Autodesk Fusion 360 part; units mm, degrees
(part 3 of 3)
  spline S561 degree 3 poles (81.8849, -47.0877) (82.1212, -46.8514) (82.4417, -46.7187) (82.7758, -46.7187) knots 0 0 0 0 1 1 1 1
  spline S562 degree 3 poles (112.4749, -35.3303) (112.8091, -35.3303) (113.1296, -35.4631) (113.3659, -35.6994) knots 0 0 0 0 1 1 1 1
  line L482 (113.7349, -36.5903) -> (113.7349, -36.5903)
  spline S563 degree 3 poles (51.3254, -35.9434) (51.2994, -35.4474) (50.8766, -35.0663) (50.3805, -35.0917) knots 0 0 0 0 1 1 1 1
  spline S564 degree 3 poles (43.0813, -29.5297) (43.3176, -29.2934) (43.6381, -29.1607) (43.9723, -29.1607) knots 0 0 0 0 1 1 1 1
  spline S565 degree 3 poles (54.9572, -31.105) (54.6231, -31.105) (54.3026, -30.9722) (54.0663, -30.7359) knots 0 0 0 0 1 1 1 1
  spline S566 degree 3 poles (51.5248, -30.1328) (51.5248, -30.6792) (51.3077, -31.2032) (50.9214, -31.5895) knots 0 0 0 0 1 1 1 1
  spline S567 degree 3 poles (43.0813, -31.3116) (42.845, -31.0753) (42.7123, -30.7549) (42.7123, -30.4207) knots 0 0 0 0 1 1 1 1
  spline S568 degree 3 poles (102.7091, -5.764) (103.0373, -6.0922) (103.2216, -6.5373) (103.2216, -7.0015) knots 0 0 0 0 1 1 1 1
  spline S569 degree 3 poles (88.275, -50.1347) (87.7287, -50.1347) (87.2047, -49.9176) (86.8184, -49.5313) knots 0 0 0 0 1 1 1 1
  spline S570 degree 3 poles (55.8482, -28.954) (56.0845, -29.1903) (56.2172, -29.5108) (56.2172, -29.845) knots 0 0 0 0 1 1 1 1
  spline S571 degree 3 poles (102.7091, -8.2389) (102.3809, -8.5671) (101.9358, -8.7515) (101.4716, -8.7515) knots 0 0 0 0 1 1 1 1
  spline S572 degree 3 poles (47.332, -19.1294) (47.358, -19.6254) (47.7808, -20.0065) (48.2768, -19.9811) knots 0 0 0 0 1 1 1 1
  spline S573 degree 3 poles (41.8226, -13.444) (41.8226, -13.1098) (41.9553, -12.7893) (42.1916, -12.553) knots 0 0 0 0 1 1 1 1
  spline S574 degree 3 poles (43.0826, -14.704) (42.7484, -14.704) (42.4279, -14.5712) (42.1916, -14.3349) knots 0 0 0 0 1 1 1 1
  spline S575 degree 3 poles (50.0317, -14.6128) (49.6454, -14.9991) (49.1214, -15.2161) (48.575, -15.2161) knots 0 0 0 0 1 1 1 1
  spline S576 degree 3 poles (71.5094, -50.5247) (71.3487, -50.2462) (71.0515, -50.0747) (70.73, -50.0747) knots 0 0 0 0 1 1 1 1
  line L483 (70.73, -50.0747) -> (69.42, -50.0747)
  spline S577 degree 3 poles (42.1916, -14.3349) (41.9553, -14.0986) (41.8226, -13.7782) (41.8226, -13.444) knots 0 0 0 0 1 1 1 1
  spline S578 degree 3 poles (48.575, -15.2161) (48.0287, -15.2161) (47.5047, -14.9991) (47.1184, -14.6128) knots 0 0 0 0 1 1 1 1
  spline S579 degree 3 poles (76.466, -45.9656) (76.2297, -46.2019) (75.9092, -46.3347) (75.575, -46.3347) knots 0 0 0 0 1 1 1 1
  spline S580 degree 3 poles (75.575, -46.3347) (75.2408, -46.3347) (74.9203, -46.2019) (74.684, -45.9656) knots 0 0 0 0 1 1 1 1
  spline S581 degree 3 poles (50.4357, -18.9667) (50.4097, -18.4707) (49.9868, -18.0896) (49.4908, -18.115) knots 0 0 0 0 1 1 1 1
  spline S582 degree 3 poles (55.3275, -12.8683) (55.3275, -13.2025) (55.1948, -13.5229) (54.9585, -13.7592) knots 0 0 0 0 1 1 1 1
  line L484 (49.585, -19.9125) -> (48.2768, -19.9811)
  spline S583 degree 3 poles (46.515, -13.1561) (46.515, -12.0184) (47.4373, -11.0961) (48.575, -11.0961) knots 0 0 0 0 1 1 1 1
  spline S584 degree 3 poles (50.0317, -11.6995) (50.418, -12.0858) (50.635, -12.6098) (50.635, -13.1561) knots 0 0 0 0 1 1 1 1
  spline S585 degree 3 poles (74.684, -45.9656) (74.4477, -45.7293) (74.315, -45.4088) (74.315, -45.0747) knots 0 0 0 0 1 1 1 1
  spline S586 degree 3 poles (70.73, -51.8747) (71.0515, -51.8747) (71.3487, -51.7031) (71.5094, -51.4247) knots 0 0 0 0 1 1 1 1
  spline S587 degree 3 poles (74.684, -44.1837) (74.9203, -43.9474) (75.2408, -43.8147) (75.575, -43.8147) knots 0 0 0 0 1 1 1 1
  spline S588 degree 3 poles (76.466, -44.1837) (76.7023, -44.42) (76.835, -44.7405) (76.835, -45.0747) knots 0 0 0 0 1 1 1 1
  spline S589 degree 3 poles (75.575, -43.8147) (75.9092, -43.8147) (76.2297, -43.9474) (76.466, -44.1837) knots 0 0 0 0 1 1 1 1
  spline S590 degree 3 poles (54.0675, -11.6083) (54.4017, -11.6083) (54.7222, -11.741) (54.9585, -11.9773) knots 0 0 0 0 1 1 1 1
  spline S591 degree 3 poles (43.0826, -12.184) (43.4168, -12.184) (43.7372, -12.3167) (43.9735, -12.553) knots 0 0 0 0 1 1 1 1
  line L485 (70.73, -51.8747) -> (69.42, -51.8747)
  spline S592 degree 3 poles (48.575, -11.0961) (49.1214, -11.0961) (49.6454, -11.3132) (50.0317, -11.6995) knots 0 0 0 0 1 1 1 1
  spline S593 degree 3 poles (53.1766, -13.7592) (52.9403, -13.5229) (52.8075, -13.2025) (52.8075, -12.8683) knots 0 0 0 0 1 1 1 1
  spline S594 degree 3 poles (53.1766, -11.9773) (53.4129, -11.741) (53.7333, -11.6083) (54.0675, -11.6083) knots 0 0 0 0 1 1 1 1
  spline S595 degree 3 poles (47.1184, -14.6128) (46.7321, -14.2264) (46.515, -13.7025) (46.515, -13.1561) knots 0 0 0 0 1 1 1 1
  spline S596 degree 3 poles (74.315, -45.0747) (74.315, -44.7405) (74.4477, -44.42) (74.684, -44.1837) knots 0 0 0 0 1 1 1 1
  line L486 (55.3275, -12.8683) -> (55.3275, -12.8683)
  spline S597 degree 3 poles (43.9735, -12.553) (44.2098, -12.7893) (44.3426, -13.1098) (44.3426, -13.444) knots 0 0 0 0 1 1 1 1
  spline S598 degree 3 poles (52.8075, -12.8683) (52.8075, -12.5341) (52.9403, -12.2136) (53.1766, -11.9773) knots 0 0 0 0 1 1 1 1
  spline S599 degree 3 poles (76.835, -45.0747) (76.835, -45.4088) (76.7023, -45.7293) (76.466, -45.9656) knots 0 0 0 0 1 1 1 1
  spline S600 degree 3 poles (68.6406, -50.5247) (68.4798, -50.8031) (68.4798, -51.1462) (68.6406, -51.4247) knots 0 0 0 0 1 1 1 1
  spline S601 degree 3 poles (72.135, -45.0747) (72.135, -45.621) (71.918, -46.145) (71.5316, -46.5313) knots 0 0 0 0 1 1 1 1
  spline S602 degree 3 poles (48.1826, -18.1836) (47.6867, -18.2101) (47.306, -18.6334) (47.332, -19.1294) knots 0 0 0 0 1 1 1 1
  spline S603 degree 3 poles (54.9585, -13.7592) (54.7222, -13.9955) (54.4017, -14.1283) (54.0675, -14.1283) knots 0 0 0 0 1 1 1 1
  line L487 (44.3426, -13.444) -> (44.3426, -13.444)
  spline S604 degree 3 poles (68.6406, -51.4247) (68.8013, -51.7031) (69.0985, -51.8747) (69.42, -51.8747) knots 0 0 0 0 1 1 1 1
  spline S605 degree 3 poles (69.42, -50.0747) (69.0985, -50.0747) (68.8013, -50.2462) (68.6406, -50.5247) knots 0 0 0 0 1 1 1 1
  spline S606 degree 3 poles (49.585, -19.9125) (50.081, -19.886) (50.4617, -19.4627) (50.4357, -18.9667) knots 0 0 0 0 1 1 1 1
  spline S607 degree 3 poles (71.5316, -46.5313) (71.1453, -46.9176) (70.6213, -47.1347) (70.075, -47.1347) knots 0 0 0 0 1 1 1 1
  spline S608 degree 3 poles (44.3426, -13.444) (44.3426, -13.7782) (44.2098, -14.0986) (43.9735, -14.3349) knots 0 0 0 0 1 1 1 1
  spline S609 degree 3 poles (68.015, -45.0747) (68.015, -43.9369) (68.9373, -43.0147) (70.075, -43.0147) knots 0 0 0 0 1 1 1 1
  spline S610 degree 3 poles (70.075, -47.1347) (69.5287, -47.1347) (69.0047, -46.9176) (68.6184, -46.5313) knots 0 0 0 0 1 1 1 1
  spline S611 degree 3 poles (54.9585, -11.9773) (55.1948, -12.2136) (55.3275, -12.5341) (55.3275, -12.8683) knots 0 0 0 0 1 1 1 1
  line L488 (72.135, -45.0747) -> (72.135, -45.0747)
  spline S612 degree 3 poles (65.835, -45.0747) (65.835, -45.4088) (65.7023, -45.7293) (65.466, -45.9656) knots 0 0 0 0 1 1 1 1
  spline S613 degree 3 poles (70.075, -43.0147) (70.6213, -43.0147) (71.1453, -43.2317) (71.5316, -43.618) knots 0 0 0 0 1 1 1 1
  spline S614 degree 3 poles (64.575, -46.3347) (64.2408, -46.3347) (63.9203, -46.2019) (63.684, -45.9656) knots 0 0 0 0 1 1 1 1
  spline S615 degree 3 poles (54.0675, -14.1283) (53.7333, -14.1283) (53.4129, -13.9955) (53.1766, -13.7592) knots 0 0 0 0 1 1 1 1
  spline S616 degree 3 poles (43.9735, -14.3349) (43.7372, -14.5712) (43.4168, -14.704) (43.0826, -14.704) knots 0 0 0 0 1 1 1 1
  spline S617 degree 3 poles (65.466, -45.9656) (65.2297, -46.2019) (64.9092, -46.3347) (64.575, -46.3347) knots 0 0 0 0 1 1 1 1
  spline S618 degree 3 poles (42.1916, -12.553) (42.4279, -12.3167) (42.7484, -12.184) (43.0826, -12.184) knots 0 0 0 0 1 1 1 1
  spline S619 degree 3 poles (71.5094, -51.4247) (71.6702, -51.1462) (71.6702, -50.8031) (71.5094, -50.5247) knots 0 0 0 0 1 1 1 1
  spline S620 degree 3 poles (68.6184, -46.5313) (68.232, -46.145) (68.015, -45.621) (68.015, -45.0747) knots 0 0 0 0 1 1 1 1
  spline S621 degree 3 poles (63.315, -45.0747) (63.315, -44.7405) (63.4477, -44.42) (63.684, -44.1837) knots 0 0 0 0 1 1 1 1
  spline S622 degree 3 poles (63.684, -45.9656) (63.4477, -45.7293) (63.315, -45.4088) (63.315, -45.0747) knots 0 0 0 0 1 1 1 1
  line L489 (49.4908, -18.115) -> (48.1826, -18.1836)
  line L490 (50.635, -13.1561) -> (50.635, -13.1561)
  line L491 (76.835, -45.0747) -> (76.835, -45.0747)
  spline S623 degree 3 poles (71.5316, -43.618) (71.918, -44.0043) (72.135, -44.5283) (72.135, -45.0747) knots 0 0 0 0 1 1 1 1
  spline S624 degree 3 poles (50.635, -13.1561) (50.635, -13.7025) (50.418, -14.2264) (50.0317, -14.6128) knots 0 0 0 0 1 1 1 1
  line L492 (65.835, -45.0747) -> (65.835, -45.0747)
  line L493 (110.7912, -73.1802) -> (111.0216, -73.8484)
  spline S625 degree 3 poles (63.684, -44.1837) (63.9203, -43.9474) (64.2408, -43.8147) (64.575, -43.8147) knots 0 0 0 0 1 1 1 1
  spline S626 degree 3 poles (3.6391, -67.1258) (4.4065, -69.4383) (6.4962, -71.0571) (8.9271, -71.2222) knots 0 0 0 0 1 1 1 1
  line L494 (116.1996, -81.9373) -> (119.0491, -76.0948)
  spline S627 degree 3 poles (118.8062, -6.1021) (83.6894, 2.7201) (46.8363, 1.8437) (12.1786, -8.6379) knots 0 0 0 0 1 1 1 1
  spline S628 degree 3 poles (118.1824, -90.992) (120.517, -91.6893) (123.0415, -90.9056) (124.5707, -89.0087) knots 0 0 0 0 1 1 1 1
  spline S629 degree 3 poles (65.466, -44.1837) (65.7023, -44.42) (65.835, -44.7405) (65.835, -45.0747) knots 0 0 0 0 1 1 1 1
  spline S630 degree 3 poles (138.6019, -30.79) (137.1962, -24.0467) (134.803, -17.5478) (131.4995, -11.5033) knots 0 0 0 0 1 1 1 1
  spline S631 degree 3 poles (64.575, -43.8147) (64.9092, -43.8147) (65.2297, -43.9474) (65.466, -44.1837) knots 0 0 0 0 1 1 1 1
  line L495 (115.2322, -66.3558) -> (114.1098, -68.657)
  line L496 (114.1098, -68.657) -> (113.6783, -68.4466)
  line L497 (111.2113, -79.5044) -> (110.0827, -81.8184)
  line L498 (115.3459, -81.5208) -> (116.1996, -81.9373)
  spline S632 degree 3 poles (124.5707, -89.0087) (128.8939, -83.6461) (132.402, -77.6748) (134.9814, -71.2878) knots 0 0 0 0 1 1 1 1
  spline S633 degree 3 poles (8.9271, -71.2222) (45.9666, -73.7356) (82.6109, -80.3665) (118.1824, -90.992) knots 0 0 0 0 1 1 1 1
  spline S634 degree 3 poles (97.4738, -79.183) (97.9614, -79.2773) (98.4333, -78.9586) (98.5281, -78.4711) knots 0 0 0 0 1 1 1 1
  spline S635 degree 3 poles (118.1954, -75.6788) (117.8944, -75.4783) (117.6795, -75.1722) (117.5933, -74.8209) knots 0 0 0 0 1 1 1 1
  line L499 (117.7292, -73.7822) -> (118.4305, -72.3441)
  line L500 (110.0827, -81.8184) -> (114.2168, -83.8348)
  line L501 (118.4305, -72.3441) -> (118.0383, -71.0961)
  spline S636 degree 3 poles (117.5933, -74.8209) (117.507, -74.4699) (117.5555, -74.0992) (117.7292, -73.7822) knots 0 0 0 0 1 1 1 1
  line L502 (114.2168, -83.8348) -> (115.3459, -81.5208)
  spline S637 degree 3 poles (139.7972, -51.3076) (140.4104, -44.4469) (140.0076, -37.5332) (138.6019, -30.79) knots 0 0 0 0 1 1 1 1
  spline S638 degree 3 poles (98.5281, -78.4711) (98.6228, -77.9835) (98.3047, -77.5113) (97.8172, -77.4161) knots 0 0 0 0 1 1 1 1
  line L503 (111.0216, -73.8484) -> (111.9203, -74.2871)
  spline S639 degree 3 poles (112.2014, -74.701) (112.2073, -74.7888) (112.1896, -74.8766) (112.1503, -74.9553) knots 0 0 0 0 1 1 1 1
  line L504 (112.1503, -74.9553) -> (110.1778, -79)
  spline S640 degree 3 poles (8.6506, -11.5033) (-0.664, -28.546) (-2.4792, -48.6926) (3.6391, -67.1258) knots 0 0 0 0 1 1 1 1
  spline S641 degree 3 poles (134.9814, -71.2878) (137.561, -64.901) (139.1837, -58.1684) (139.7972, -51.3076) knots 0 0 0 0 1 1 1 1
  line L505 (112.9833, -68.6859) -> (110.7912, -73.1802)
  spline S642 degree 3 poles (131.4995, -11.5033) (130.7448, -10.1225) (129.4778, -9.0934) (127.9715, -8.6379) knots 0 0 0 0 1 1 1 1
  line L506 (110.1778, -79) -> (111.2113, -79.5044)
  line L507 (119.3664, -68.3727) -> (115.2322, -66.3558)
  line L508 (115.2322, -66.3558) -> (115.2322, -66.3558)
  spline S643 degree 3 poles (112.1172, -74.4556) (112.1666, -74.5284) (112.1957, -74.6132) (112.2014, -74.701) knots 0 0 0 0 1 1 1 1
  line L509 (113.6783, -68.4466) -> (112.9833, -68.6859)
  line L510 (119.0491, -76.0948) -> (118.1954, -75.6788)
  spline S644 degree 3 poles (111.9203, -74.2871) (111.9997, -74.3248) (112.0677, -74.3829) (112.1172, -74.4556) knots 0 0 0 0 1 1 1 1
  spline S645 degree 3 poles (12.1786, -8.6379) (10.6723, -9.0934) (9.4054, -10.1225) (8.6506, -11.5033) knots 0 0 0 0 1 1 1 1
  line L511 (118.0383, -71.0961) -> (119.3664, -68.3727)
  spline S646 degree 3 poles (74.315, -11.0747) (74.315, -10.7405) (74.4477, -10.42) (74.684, -10.1837) knots 0 0 0 0 1 1 1 1
  line L512 (72.135, -11.0747) -> (72.135, -11.0747)
  spline S647 degree 3 poles (40.9202, -28.6515) (41.5169, -28.6515) (42.0892, -28.8885) (42.5112, -29.3105) knots 0 0 0 0 1 1 1 1
  spline S648 degree 3 poles (59.9702, -9.6015) (60.5669, -9.6015) (61.1392, -9.8385) (61.5612, -10.2605) knots 0 0 0 0 1 1 1 1
  line L513 (73.095, -19.3947) -> (73.095, -19.8747)
  line L514 (65.835, -11.0747) -> (65.835, -11.0747)
  spline S649 degree 3 poles (57.7202, -11.8515) (57.7202, -11.2547) (57.9573, -10.6824) (58.3792, -10.2605) knots 0 0 0 0 1 1 1 1
  line L515 (118.8062, -6.1023) -> (117.075, -12.3447)
  spline S650 degree 3 poles (63.684, -11.9656) (63.4477, -11.7293) (63.315, -11.4088) (63.315, -11.0747) knots 0 0 0 0 1 1 1 1
  spline S651 degree 3 poles (70.075, -9.0147) (70.6213, -9.0147) (71.1453, -9.2317) (71.5316, -9.618) knots 0 0 0 0 1 1 1 1
  spline S652 degree 3 poles (65.835, -11.0747) (65.835, -11.4088) (65.7023, -11.7293) (65.466, -11.9656) knots 0 0 0 0 1 1 1 1
  spline S653 degree 3 poles (70.075, -13.1347) (69.5287, -13.1347) (69.0047, -12.9176) (68.6184, -12.5313) knots 0 0 0 0 1 1 1 1
  spline S654 degree 3 poles (63.315, -11.0747) (63.315, -10.7405) (63.4477, -10.42) (63.684, -10.1837) knots 0 0 0 0 1 1 1 1
  line L516 (86.2116, -49.5825) -> (86.2116, -52.9465)
  spline S655 degree 3 poles (43.1702, -30.9015) (43.1702, -31.4982) (42.9331, -32.0705) (42.5112, -32.4925) knots 0 0 0 0 1 1 1 1
  spline S656 degree 3 poles (39.3292, -32.4925) (38.9073, -32.0705) (38.6702, -31.4982) (38.6702, -30.9015) knots 0 0 0 0 1 1 1 1
  line L517 (70.73, -17.8747) -> (69.42, -17.8747)
  spline S657 degree 3 poles (61.5612, -10.2605) (61.9831, -10.6824) (62.2202, -11.2547) (62.2202, -11.8515) knots 0 0 0 0 1 1 1 1
  line L518 (43.1702, -30.9015) -> (43.1702, -30.9015)
  line L519 (78.8459, -52.9465) -> (78.8459, -49.5825)
  line L520 (73.095, -19.8747) -> (75.655, -19.8747)
  spline S658 degree 3 poles (58.3792, -10.2605) (58.8012, -9.8385) (59.3735, -9.6015) (59.9702, -9.6015) knots 0 0 0 0 1 1 1 1
  line L521 (68.575, -27.5747) -> (68.575, -26.6247)
  line L522 (67.075, -20.3747) -> (67.075, -19.3747)
  spline S659 degree 3 poles (71.5316, -9.618) (71.918, -10.0043) (72.135, -10.5283) (72.135, -11.0747) knots 0 0 0 0 1 1 1 1
  line L523 (62.075, -27.5747) -> (62.075, -26.6247)
  spline S660 degree 3 poles (59.9702, -14.1015) (59.3735, -14.1015) (58.8012, -13.8644) (58.3792, -13.4425) knots 0 0 0 0 1 1 1 1
  spline S661 degree 3 poles (75.575, -9.8147) (75.9092, -9.8147) (76.2297, -9.9474) (76.466, -10.1837) knots 0 0 0 0 1 1 1 1
  spline S662 degree 3 poles (68.6184, -12.5313) (68.232, -12.145) (68.015, -11.621) (68.015, -11.0747) knots 0 0 0 0 1 1 1 1
  line L524 (86.2116, -52.9465) -> (78.8459, -52.9465)
  spline S663 degree 3 poles (74.684, -10.1837) (74.9203, -9.9474) (75.2408, -9.8147) (75.575, -9.8147) knots 0 0 0 0 1 1 1 1
  spline S664 degree 3 poles (65.466, -11.9656) (65.2297, -12.2019) (64.9092, -12.3347) (64.575, -12.3347) knots 0 0 0 0 1 1 1 1
  line L525 (78.8459, -49.5825) -> (86.2116, -49.5825)
  spline S665 degree 3 poles (70.075, -25.3747) (69.3264, -25.3389) (68.6749, -25.8819) (68.575, -26.6247) knots 0 0 0 0 1 1 1 1
  line L526 (62.2202, -11.8515) -> (62.2202, -11.8515)
  spline S666 degree 3 poles (76.466, -10.1837) (76.7023, -10.42) (76.835, -10.7405) (76.835, -11.0747) knots 0 0 0 0 1 1 1 1
  line L527 (126.0175, -14.8246) -> (127.7516, -8.5716)
  spline S667 degree 3 poles (64.575, -12.3347) (64.2408, -12.3347) (63.9203, -12.2019) (63.684, -11.9656) knots 0 0 0 0 1 1 1 1
  spline S668 degree 3 poles (64.575, -9.8147) (64.9092, -9.8147) (65.2297, -9.9474) (65.466, -10.1837) knots 0 0 0 0 1 1 1 1
  spline S669 degree 3 poles (63.684, -10.1837) (63.9203, -9.9474) (64.2408, -9.8147) (64.575, -9.8147) knots 0 0 0 0 1 1 1 1
  spline S670 degree 3 poles (65.466, -10.1837) (65.7023, -10.42) (65.835, -10.7405) (65.835, -11.0747) knots 0 0 0 0 1 1 1 1
  spline S671 degree 3 poles (61.5612, -13.4425) (61.1392, -13.8644) (60.5669, -14.1015) (59.9702, -14.1015) knots 0 0 0 0 1 1 1 1
  spline S672 degree 3 poles (38.6702, -30.9015) (38.6702, -30.3047) (38.9073, -29.7324) (39.3292, -29.3105) knots 0 0 0 0 1 1 1 1
  spline S673 degree 3 poles (66.575, -20.8747) (66.708, -20.876) (66.836, -20.8238) (66.9301, -20.7297) knots 0 0 0 0 1 1 1 1
  spline S674 degree 3 poles (39.3292, -29.3105) (39.7512, -28.8885) (40.3235, -28.6515) (40.9202, -28.6515) knots 0 0 0 0 1 1 1 1
  spline S675 degree 3 poles (71.5316, -12.5313) (71.1453, -12.9176) (70.6213, -13.1347) (70.075, -13.1347) knots 0 0 0 0 1 1 1 1
  spline S676 degree 3 poles (40.9202, -33.1515) (40.3235, -33.1515) (39.7512, -32.9144) (39.3292, -32.4925) knots 0 0 0 0 1 1 1 1
  line L528 (117.075, -12.3447) -> (126.0175, -14.8246)
  line L529 (68.575, -27.5747) -> (62.075, -27.5747)
  spline S677 degree 3 poles (42.5112, -32.4925) (42.0892, -32.9144) (41.5169, -33.1515) (40.9202, -33.1515) knots 0 0 0 0 1 1 1 1
  spline S678 degree 3 poles (42.5112, -29.3105) (42.9331, -29.7324) (43.1702, -30.3047) (43.1702, -30.9015) knots 0 0 0 0 1 1 1 1
  spline S679 degree 3 poles (72.135, -11.0747) (72.135, -11.621) (71.918, -12.145) (71.5316, -12.5313) knots 0 0 0 0 1 1 1 1
  spline S680 degree 3 poles (66.9301, -20.7297) (67.0241, -20.6356) (67.0764, -20.5077) (67.075, -20.3747) knots 0 0 0 0 1 1 1 1
  line L530 (72.575, -18.8747) -> (73.095, -19.3947)
  spline S681 degree 3 poles (62.2202, -11.8515) (62.2202, -12.4482) (61.9831, -13.0205) (61.5612, -13.4425) knots 0 0 0 0 1 1 1 1
  line L531 (62.075, -22.0247) -> (62.075, -20.8747)
  spline S682 degree 3 poles (58.3792, -13.4425) (57.9573, -13.0205) (57.7202, -12.4482) (57.7202, -11.8515) knots 0 0 0 0 1 1 1 1
  line L532 (76.835, -11.0747) -> (76.835, -11.0747)
  spline S683 degree 3 poles (68.015, -11.0747) (68.015, -9.9369) (68.9373, -9.0147) (70.075, -9.0147) knots 0 0 0 0 1 1 1 1
  spline S684 degree 3 poles (104.9284, -54.8447) (104.542, -54.4584) (104.325, -53.9344) (104.325, -53.388) knots 0 0 0 0 1 1 1 1
  spline S685 degree 3 poles (100.8883, -54.4561) (100.1925, -54.4561) (99.6283, -53.892) (99.6283, -53.1961) knots 0 0 0 0 1 1 1 1
  spline S686 degree 3 poles (100.8883, -51.9361) (101.2225, -51.9361) (101.543, -52.0688) (101.7793, -52.3051) knots 0 0 0 0 1 1 1 1
  spline S687 degree 3 poles (107.7325, -59.3387) (107.7498, -58.8422) (107.3616, -58.4255) (106.8651, -58.4079) knots 0 0 0 0 1 1 1 1
  line L533 (62.075, -20.8747) -> (66.575, -20.8747)
  spline S688 degree 3 poles (68.6406, -17.4247) (68.8013, -17.7031) (69.0985, -17.8747) (69.42, -17.8747) knots 0 0 0 0 1 1 1 1
  line L534 (71.675, -25.3747) -> (70.075, -25.3747)
  line L535 (75.655, -24.4747) -> (75.655, -19.8747)
  spline S689 degree 3 poles (76.466, -11.9656) (76.2297, -12.2019) (75.9092, -12.3347) (75.575, -12.3347) knots 0 0 0 0 1 1 1 1
  spline S690 degree 3 poles (71.5094, -17.4247) (71.6702, -17.1462) (71.6702, -16.8031) (71.5094, -16.5247) knots 0 0 0 0 1 1 1 1
  line L536 (67.575, -18.8747) -> (72.575, -18.8747)
  line L537 (72.625, -24.4747) -> (71.675, -25.3747)
  spline S691 degree 3 poles (71.5094, -16.5247) (71.3487, -16.2462) (71.0515, -16.0747) (70.73, -16.0747) knots 0 0 0 0 1 1 1 1
  spline S692 degree 3 poles (74.684, -11.9656) (74.4477, -11.7293) (74.315, -11.4088) (74.315, -11.0747) knots 0 0 0 0 1 1 1 1
  line L538 (70.73, -16.0747) -> (69.42, -16.0747)
  line L539 (104.7873, -73.4324) -> (104.7873, -73.4324)
  spline S693 degree 3 poles (100.1883, -72.3829) (100.1883, -73.5206) (99.266, -74.4429) (98.1283, -74.4429) knots 0 0 0 0 1 1 1 1
  spline S694 degree 3 poles (96.6717, -73.8396) (96.2853, -73.4533) (96.0683, -72.9293) (96.0683, -72.3829) knots 0 0 0 0 1 1 1 1
  line L540 (62.075, -26.6247) -> (59.5, -26.6247)
  spline S695 degree 3 poles (103.5273, -72.1724) (103.8614, -72.1724) (104.1819, -72.3051) (104.4182, -72.5414) knots 0 0 0 0 1 1 1 1
  spline S696 degree 3 poles (98.1283, -74.4429) (97.582, -74.4429) (97.058, -74.2259) (96.6717, -73.8396) knots 0 0 0 0 1 1 1 1
  line L541 (100.1883, -72.3829) -> (100.1883, -72.3829)
  spline S697 degree 3 poles (106.8023, -60.2068) (107.2988, -60.2237) (107.7152, -59.8352) (107.7325, -59.3387) knots 0 0 0 0 1 1 1 1
  line L542 (59.5, -22.0247) -> (62.075, -22.0247)
  spline S698 degree 3 poles (105.5559, -58.3621) (105.0594, -58.3451) (104.643, -58.7337) (104.6257, -59.2302) knots 0 0 0 0 1 1 1 1
  spline S699 degree 3 poles (108.445, -53.388) (108.445, -53.9344) (108.228, -54.4584) (107.8416, -54.8447) knots 0 0 0 0 1 1 1 1
  spline S700 degree 3 poles (104.6257, -59.2302) (104.6083, -59.7267) (104.9966, -60.1433) (105.4931, -60.161) knots 0 0 0 0 1 1 1 1
  line L543 (106.8023, -60.2068) -> (105.4931, -60.161)
  spline S701 degree 3 poles (107.8416, -54.8447) (107.4553, -55.231) (106.9313, -55.448) (106.385, -55.448) knots 0 0 0 0 1 1 1 1
  spline S702 degree 3 poles (104.9284, -51.9314) (105.3147, -51.5451) (105.8387, -51.328) (106.385, -51.328) knots 0 0 0 0 1 1 1 1
  spline S703 degree 3 poles (106.385, -51.328) (106.9313, -51.328) (107.4553, -51.5451) (107.8416, -51.9314) knots 0 0 0 0 1 1 1 1
  spline S704 degree 3 poles (76.835, -11.0747) (76.835, -11.4088) (76.7023, -11.7293) (76.466, -11.9656) knots 0 0 0 0 1 1 1 1
  line L544 (108.445, -53.388) -> (108.445, -53.388)
  spline S705 degree 3 poles (101.7793, -54.087) (101.543, -54.3233) (101.2225, -54.4561) (100.8883, -54.4561) knots 0 0 0 0 1 1 1 1
  spline S706 degree 3 poles (104.325, -53.388) (104.325, -52.8417) (104.542, -52.3177) (104.9284, -51.9314) knots 0 0 0 0 1 1 1 1
  spline S707 degree 3 poles (70.73, -17.8747) (71.0515, -17.8747) (71.3487, -17.7031) (71.5094, -17.4247) knots 0 0 0 0 1 1 1 1
  spline S708 degree 3 poles (75.575, -12.3347) (75.2408, -12.3347) (74.9203, -12.2019) (74.684, -11.9656) knots 0 0 0 0 1 1 1 1
  spline S709 degree 3 poles (102.6363, -72.5414) (102.8726, -72.3051) (103.1931, -72.1724) (103.5273, -72.1724) knots 0 0 0 0 1 1 1 1
  line L545 (67.075, -19.3747) -> (67.575, -18.8747)
  line L546 (75.655, -24.4747) -> (72.625, -24.4747)
  spline S710 degree 3 poles (96.6717, -70.9263) (97.058, -70.54) (97.582, -70.3229) (98.1283, -70.3229) knots 0 0 0 0 1 1 1 1
  line L547 (59.5, -26.6247) -> (59.5, -22.0247)
  spline S711 degree 3 poles (98.1283, -70.3229) (99.266, -70.3229) (100.1883, -71.2452) (100.1883, -72.3829) knots 0 0 0 0 1 1 1 1
  line L548 (106.8651, -58.4079) -> (105.5559, -58.3621)
  spline S712 degree 3 poles (106.385, -55.448) (105.8387, -55.448) (105.3147, -55.231) (104.9284, -54.8447) knots 0 0 0 0 1 1 1 1
  spline S713 degree 3 poles (107.8416, -51.9314) (108.228, -52.3177) (108.445, -52.8417) (108.445, -53.388) knots 0 0 0 0 1 1 1 1
  spline S714 degree 3 poles (69.42, -16.0747) (69.0985, -16.0747) (68.8013, -16.2462) (68.6406, -16.5247) knots 0 0 0 0 1 1 1 1
  spline S715 degree 3 poles (104.4182, -72.5414) (104.6545, -72.7777) (104.7873, -73.0982) (104.7873, -73.4324) knots 0 0 0 0 1 1 1 1
  spline S716 degree 3 poles (102.1483, -53.1961) (102.1483, -53.5303) (102.0156, -53.8508) (101.7793, -54.087) knots 0 0 0 0 1 1 1 1
  spline S717 degree 3 poles (68.6406, -16.5247) (68.4798, -16.8031) (68.4798, -17.1462) (68.6406, -17.4247) knots 0 0 0 0 1 1 1 1
  spline S718 degree 3 poles (96.0683, -72.3829) (96.0683, -71.8366) (96.2853, -71.3126) (96.6717, -70.9263) knots 0 0 0 0 1 1 1 1
extrude "Extrude2" add sketch "Sketch1" along normal blind 1 from surface at 3 contours S0 S14 S23 S43 S179 S180 L362 S181 L365 L366 L367 L368 L372 L381 L382 L383 L384 L385 L390 L394 L396 L398 L399 L400 L403 S710 S718 | S7 S44 L255 L258 L260 L262 L263 L264 L265 L266 L267 L268 L270 L271 L276 L277 L380 S194 L388 L389 L391 S217 S224 S686 S702 S706 | S18 S22 S50 S233 S237 L406 L408 L409 L410 L412 L413 L414 L415 L417 L418 S250 L422 L423 L424 L425 L426 L428 S278 S290 S299 S314 S318 | S25 S32 S37 L8 L10 L13 L16 L34 L35 L39 L40 L41 L42 L43 L44 L48 L49 L54 L56 L59 L65 S373 S379 S380 S383 S396 | L14 S51 L17 L18 L25 L27 L29 L30 L31 L32 L36 L45 S59 L55 L57 L58 L60 S61 L62 L63 L64 S265 S267 S297 S310 S316 | L15 L19 L20 L21 L22 L23 L26 L28 L33 L37 L38 L46 L47 L50 L51 L52 S57 S58 L53 S60 L93 S208 S209 S210 S220 S221 | S62 L66 L67 S63 L68 L69 L70 S65 L72 L73 L74 L75 L80 L81 L89 L94 L95 L98 L99 L101 L106 S464 S471 S494 S504 S511 S517 | L78 L79 L84 L85 L86 S74 L87 L88 L90 L91 L92 S76 L96 S77 L100 L102 L103 L104 L105 L116 L142 L154 S469 S473 S478 S479 S500 S507 | S79 L111 S82 L112 L113 L114 S83 L115 L117 S87 L119 L121 L125 L127 S90 L134 L136 L137 L139 L140 L146 L148 L149 S334 S370 S389 S390 S397 S406 S407 L493 L494 L495 L496 L497 L498 S635 L499 L500 L501 S636 L502 L503 S639 L504 L505 L506 L507 S643 L509 L510 S644 L511 | L110 S81 L118 L120 L126 S89 L129 S91 L141 L143 L144 L145 L313 L316 L321 L322 L324 L325 L326 L327 L330 S519 S539 S553 S555 S561 | S93 L208 L209 S94 L212 L213 L214 L217 L218 L219 L220 L221 L222 L223 L224 L225 L226 L227 L231 L232 S98 S420 S421 S427 S448 S456 | S112 S113 L238 L240 L241 L243 L245 L246 L247 L248 L249 L250 L251 L252 L253 L254 L256 L257 L259 S118 L261 S324 S331 S346 S352 S356 | S117 S119 L269 L272 L273 L274 L275 L278 S122 L282 L283 L285 L287 L288 S127 L290 L292 S130 L295 S131 S132 S133 S135 S136 L296 L297 L298 L300 S157 S648 S654 S658 S668 S669 S670 S683 | L301 S140 L303 L305 L308 L309 S150 L310 L311 L312 L314 L315 S158 L318 L319 L320 L328 L329 L331 L332 S532 S537 S540 S551 S564 S647 S674 S678 | S143 S163 L334 L336 L337 L338 S174 L340 L341 L342 L344 L351 L356 L357 L358 L360 L363 L364 L373 L374 L375 S573 S583 S591 S597 S618 | L333 L335 L339 L346 S175 L347 L348 L350 L352 L353 L354 L355 L359 L361 S185 L370 L371 L376 S189 L377 L378 S609 S621 S625 S629 S631 | S449 S450 S455 S460 S466 L513 L520 L521 L522 L523 S665 S673 L529 S680 L530 L531 L533 L534 L535 L536 L537 L540 L542 L545 L546 L547 makes body 1 at (106.5951, -47.2521, 3) makes body 2 at (50.029, -40.9787, 3) makes body 3 at (107.7817, -13.2729, 3) makes body 4 at (49.1393, -24.002, 3) makes body 5 at (30.1722, -33.3266, 3) makes body 6 at (88.9714, -7.9412, 3) makes body 7 at (70.0708, -21.9352, 3) makes body 8 at (88.378, -41.936, 3) makes body 9 at (99.2979, -66.3518, 3) makes body 10 at (31.6539, -50.2619, 3) makes body 11 at (107.1884, -30.2625, 3) makes body 12 at (48.2496, -7.0253, 3) makes body 13 at (12.2407, -34.8954, 3) makes body 14 at (64.4635, -6.2416, 3) makes body 15 at (88.6747, -24.9386, 3) makes body 16 at (70.0708, -38.9352, 3) makes body 17 at (113.3383, -77.9133, 3)
extrude "Extrude1" add sketch "Sketch1" along normal blind 4 separate body contours L78 L79 L84 L85 L86 S74 L87 L88 L90 L91 L92 S76 L96 S77 L100 L102 L103 L104 L105 L116 L130 L131 L135 L138 L142 L154 L155 L160 L166 L170 L171 L172 L173 L174 L176 L177 L178 L179 L180 L181 L182 L184 L186 L187 L188 L190 L192 L193 L194 L195 L198 L200 L201 L210 S467 S469 S470 S473 S476 S478 S487 S491 S492 S495 S498 S506 S507 S514 S626 S627 S628 S630 S632 S633 S637 S640 S641 S642 S645 | L284 L294 L516 L519 L524 L525 makes body 18
extrude "Extrude3" add sketch "Sketch1" along normal blind 0.5 from surface at 3.5 contours L78 L87 L154 L160 L166 L178 | L78 L87 L154 | L154 L159 L160 L166 | S86 L154 L159 L160 L166 L182 L184 S627 S642 L515 L527 L528 | S85 L515 L527 L528 | L135 L177 L210 S630 | L130 L155 L170 L187 L188 L192 L193 L200 L201 S637 S641 | L130 L155 L170 L187 L188 L193 L201 | L130 L131 L153 L155 L161 L170 L172 L173 L176 L179 L180 L181 L186 L187 L188 L193 L194 L195 L196 L201 | L138 L171 L173 L186 L190 L198 L201 | L161 L173 L179 L186 L190 L195 L198 L201 | L131 L172 L174 L176 L180 L181 L194 | L131 L153 L172 L176 L180 L181 L194 L196 | L107 L108 L123 L124 L133 L150 L151 | L132 L158 L162 L175 L189 L191 L197 | L156 L157 L202 L205 L206 L215 L229 | L163 L164 L167 L169 L203 L216 L233 | L165 L168 L183 L204 L207 L211 L230 bodies 18 3
